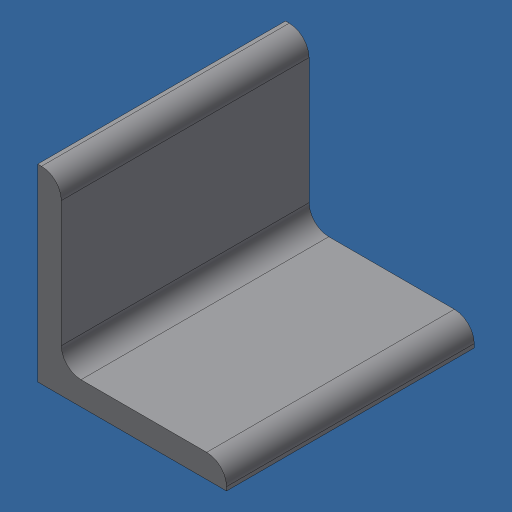
# Autodesk Inventor part: ANGLE IRON, 3 X 3 X 0.375 THK
Saved by Autodesk Inventor 2024.3 (Build 283343000, 343)
## iProperties
Category: _
Manager: _
Created: 2023-11-08
Part Number: ANGLE IRON, 3 X 3 X 0.375 THK
Checked By: 00
Engr Approved By: _
User Status: Work In Process
Material: Angle Iron
Description: ANGLE IRON, 3 X 3 X 0.375 THK
Document SubType Name: Modeling
Mfg Approved By: Stephen.Oerton
Designer: -
Mass: 1058.69 g
Surface Area: 321.464 cm^2
Volume: 134.693 cm^3
Density: 7.86 g/cm^3
Appearance: Grey (Light)
ILogicPurgeVersion: 2.2.20.20
OnSaveVersion: 2.2.20.20
CN_MASS: 1.06
CN_SERVICEABLE: _
CL_runCount: 0
FIRST_DESCRIPTION: _
SECOND_DESCRIPTION: _
THIRD_DESCRIPTION: _
ModelCat: Uncategorized
Subject: _
Author: -
Keywords: -
Revision Number: A
Autodesk Inventor part; units mm, degrees
ref_plane "YZ Plane" through (0, 0, 0) normal (1, 0, 0) x (0, 1, 0)
ref_plane "XZ Plane" through (0, 0, 0) normal (0, 1, 0) x (-1, 0, 0)
ref_plane "XY Plane" through (0, 0, 0) normal (0, 0, 1) x (1, 0, 0)
sketch "Sketch1" plane through (0, 0, 0) normal (0, 0, 1) x (1, 0, 0)
  line L0 (0, 0) -> (0, 76.2)
  line L1 (0, 76.2) -> (1.524, 76.2)
  line L2 (9.525, 68.199) -> (9.525, 17.4625)
  line L3 (0, 0) -> (76.2, 0)
  line L4 (76.2, 0) -> (76.2, 1.524)
  line L5 (68.199, 9.525) -> (17.4625, 9.525)
  arc A0 (9.525, 17.4625) -> (17.4625, 9.525) centre (17.4625, 17.4625) ccw
  arc A1 (9.525, 68.199) -> (1.524, 76.2) centre (1.524, 68.199) ccw
  arc A2 (76.2, 1.524) -> (68.199, 9.525) centre (68.199, 1.524) ccw
  dimension "thickness" = 9.525
  dimension "d3" = 9.525
  dimension "LegSize" = 76.2
  dimension "d5" = 76.2
  dimension "radius" = 7.9375
  dimension "d7" = 8.001
  dimension "d8" = 8.001
  constraints: 12 end point, 6 point on circle, 6 tangent, 4 parallel, 3 centre point, 1 coincident, 1 perpendicular, 1 vertical
  measures "thickness" distance between parallel lines of L2 L0
  measures "d3" distance between parallel lines of L5 L3
  measures "LegSize" distance of L0.start L0.end
  measures "d5" distance of L0.start L3.end
  measures "radius" radius of A0
  measures "d7" radius of A1
  measures "d8" radius of A2
extrude "3\" X 3\" X 3/8\"" add sketch "Sketch1" along normal mid plane 100
equation "\"d3\" = thickness"
equation "\"d5\" = LegSize"
